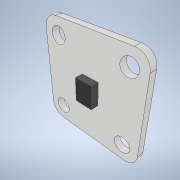
# Autodesk Inventor part: AS5600
Saved by Autodesk Inventor 2021.1 (Build 251245010, 245A)
## iProperties
Created: 2025-05-29
Part Number: AS5600
Material: Типовые
Document SubType Name: Modeling
Designer: Андрей Тарасов
Density: 1 g/cm^3
Appearance: По умолчанию
Author: Андрей Тарасов
Autodesk Inventor part; units mm, degrees
ref_plane "YZ Plane" through (0, 0, 0) normal (1, 0, 0) x (0, 1, 0)
ref_plane "XZ Plane" through (0, 0, 0) normal (0, 1, 0) x (-1, 0, 0)
ref_plane "XY Plane" through (0, 0, 0) normal (0, 0, 1) x (1, 0, 0)
sketch "Эскиз1" plane through (0, 0, 0) normal (0, 0, 1) x (1, 0, 0)
  line L0 (8.5, -11.5) -> (-8.5, -11.5)
  line L1 (-11.5, -8.5) -> (-11.5, 8.5)
  line L2 (-8.5, 11.5) -> (8.5, 11.5)
  line L3 (11.5, 8.5) -> (11.5, -8.5)
  line L4 (11.5, -11.5) -> (-11.5, 11.5) construction
  line L5 (-11.5, -11.5) -> (11.5, 11.5) construction
  line L6 (8, -8) -> (-8, -8) construction
  line L7 (-8, -8) -> (-8, 8) construction
  line L8 (-8, 8) -> (8, 8) construction
  line L9 (8, 8) -> (8, -8) construction
  line L10 (8, -8) -> (-8, 8) construction
  line L11 (-8, -8) -> (8, 8) construction
  circle A0 centre (-8, 8) radius 1.8
  circle A1 centre (8, 8) radius 1.8
  circle A2 centre (-8, -8) radius 1.8
  circle A3 centre (8, -8) radius 1.8
  arc A4 (-8.5, 11.5) -> (-11.5, 8.5) centre (-8.5, 8.5) ccw
  arc A5 (11.5, 8.5) -> (8.5, 11.5) centre (8.5, 8.5) ccw
  arc A6 (8.5, -11.5) -> (11.5, -8.5) centre (8.5, -8.5) ccw
  arc A7 (-11.5, -8.5) -> (-8.5, -11.5) centre (-8.5, -8.5) ccw
  point P0 (0, 0)
  dimension "d0" = 23
  dimension "d1" = 23
  dimension "d2" = 16
  dimension "d3" = 16
  dimension "d4" = 3.6
  dimension "d5" = 3.6
  dimension "d6" = 3.6
  dimension "d7" = 3.6
  dimension "d8" = 3
  constraints: 24 end point, 8 centre point, 8 point on circle, 8 point on line, 8 tangent, 4 coincident, 4 midpoint, 4 parallel, 3 equal radius, 2 horizontal, 2 perpendicular
  measures "d0" distance of L4.end L5.end
  measures "d1" distance of L5.start L4.end
  measures "d2" distance of L7.end L8.end
  measures "d3" distance of L6.end L7.end
  measures "d4" diameter of A0
  measures "d5" diameter of A1
  measures "d6" diameter of A2
  measures "d7" diameter of A3
  measures "d8" radius of A4
extrude "Выдавливание1" add sketch "Эскиз1" along normal blind 1.6
sketch "Эскиз2" plane through (0, 0, 1.6) normal (0, 0, 1) x (1, 0, 0)
  line L0 (-1.95, -2.5) -> (1.95, -2.5)
  line L1 (1.95, -2.5) -> (1.95, 2.5)
  line L2 (1.95, 2.5) -> (-1.95, 2.5)
  line L3 (-1.95, 2.5) -> (-1.95, -2.5)
  line L4 (-1.95, -2.5) -> (1.95, 2.5) construction
  line L5 (1.95, -2.5) -> (-1.95, 2.5) construction
  point P0 (0, 0)
  dimension "d11" = 3.9
  dimension "d12" = 5
  constraints: 12 end point, 2 midpoint, 2 parallel, 1 horizontal, 1 perpendicular
  measures "d11" distance of L2.end L1.end
  measures "d12" distance of L1.end L0.end
extrude "Выдавливание2" add sketch "Эскиз2" along normal blind 1.7
equation "\"d3\" = d2"
